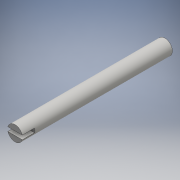
# Autodesk Inventor part: Pieza4
Saved by Autodesk Inventor 2016 (Build 200138000, 138)
## iProperties
Created: 2016-10-17
Part Number: Pieza4
Material: Genérico
Document SubType Name: Modeling
Designer: Roberto
Density: 1 g/cm^3
Appearance: Valor por defecto
Author: Roberto
Autodesk Inventor part; units mm, degrees
ref_plane "YZ Plane" through (0, 0, 0) normal (1, 0, 0) x (0, 1, 0)
ref_plane "XZ Plane" through (0, 0, 0) normal (0, 1, 0) x (-1, 0, 0)
ref_plane "XY Plane" through (0, 0, 0) normal (0, 0, 1) x (1, 0, 0)
sketch "Boceto1" plane through (0, 0, 0) normal (0, 1, 0) x (-1, 0, 0)
  circle A0 centre (0, 0) radius 0.37
  dimension "d0" = 0.74
  constraints: 1 centre point, 1 coincident
  measures "d0" diameter of A0
extrude "Extrusión1" add sketch "Boceto1" along normal blind 7.4
sketch "Boceto2" plane through (0, 0, 0) normal (0, -1, 0) x (1, 0, 0)
  line L0 (0, 0) -> (-0.6417, 0)
  line L1 (-0.6417, 0) -> (-0.6417, 0.1)
  line L2 (-0.6417, 0.1) -> (2.3583, 0.1)
  line L3 (2.3583, 0.1) -> (2.3583, -0.1)
  line L4 (2.3583, -0.1) -> (-0.6417, -0.1)
  line L5 (-0.6417, 0) -> (-0.6417, -0.1)
  dimension "d3" = 0.1
  dimension "d4" = 3
  dimension "d5" = 0.2
  constraints: 12 end point, 3 perpendicular, 2 vertical, 1 horizontal
  measures "d3" distance of L0.end L1.end
  measures "d4" distance of L1.end L2.end
  measures "d5" distance of L2.end L3.end
extrude "Extrusión2" cut sketch "Boceto2" against normal blind 0.6
